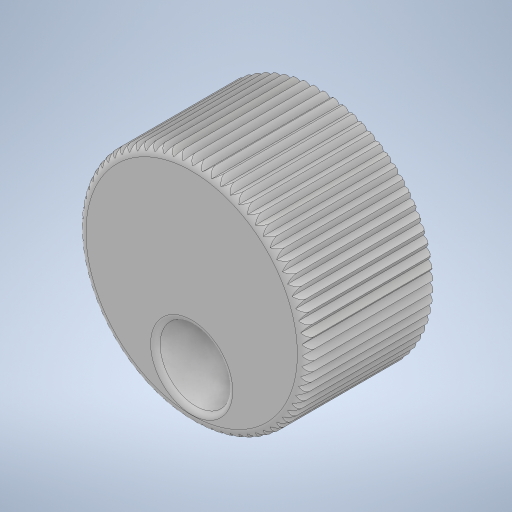
# Autodesk Inventor part: Encoder Knob
Saved by Autodesk Inventor 2024 (Build 280153000, 153)
## iProperties
Created: 2025-11-01
Part Number: Encoder Knob
Material: Generic
Document SubType Name: Modeling
Designer: Martin
Density: 1 g/cm^3
Appearance: Default
Author: Martin
Autodesk Inventor part; units mm, degrees
sketch "Sketch1" plane through (0, 0, 0) normal (0, 0, 1) x (1, 0, 0)
  circle A0 centre (0, 0) radius 15.875
  dimension "d0" = 31.75
  constraints: 1 centre point, 1 coincident
  measures "d0" diameter of A0
extrude "Extrusion1" add sketch "Sketch1" along normal blind 2.54
sketch "Sketch2" plane through (0, 0, 0) normal (0, 0, -1) x (-1, 0, 0)
  circle A0 centre (0, 0) radius 3.005
  circle A1 centre (0, 0) radius 5.08
  line L0 (0.7937, -5.0176) -> (0.7937, -2.8983)
  line L1 (-0.7937, -5.0176) -> (-0.7937, -2.8983)
  line L2 (-0.7937, -2.8983) -> (0.7937, -2.8983) construction
  line L3 (-2.6067, -1.495) -> (2.6067, -1.495) construction
  line L4 (2.5097, -1.6527) -> (2.1715, -1.495)
  line L5 (0.3685, -1.495) -> (1.9904, -2.2513)
  line L6 (0.3685, -1.495) -> (2.1715, -1.495)
  line L7 (0, -1.495) -> (0, -2.8983) construction
  line L8 (-2.5097, -1.6527) -> (-2.1715, -1.495)
  line L9 (-0.3685, -1.495) -> (-1.9904, -2.2513)
  line L10 (-0.3685, -1.495) -> (-2.1715, -1.495)
  point P0 (1.27, -1.495)
  point P1 (-1.27, -1.495)
  point P2 (-2.5097, -1.6527)
  point P3 (-1.9904, -2.2513)
  dimension "d3" = 6.01
  dimension "d4" = 10.16
  dimension "d5" = 1.5875
  dimension "d6" = 4.5
  dimension "d7" = 0.762
  dimension "d9" = 1.27
  dimension "d10" = 25
  constraints: 22 end point, 8 point on circle, 5 symmetric about line, 3 midpoint, 2 centre point, 2 coincident, 2 horizontal, 2 parallel, 2 point on line, 1 collinear, 1 vertical
  measures "d3" diameter of A0
  measures "d4" diameter of A1
  measures "d5" distance between parallel lines of L0 L1
  measures "d7" distance between parallel lines of L5 L4
  measures "d9" distance of L7.start point (1.27, -1.495)
  measures "d10" angle of L5 L3
extrude "Extrusion2" add sketch "Sketch2" along normal blind 6.35 contours A0 L1 A1 L0 | L8 L10 L9 A0 | A0 L5 L6 L4 picked at (4.3399, 0.4021)
sketch "Sketch3" plane through (0, 0, 0) normal (0, 0, -1) x (-1, 0, 0)
  circle A0 centre (0, 0) radius 15.875 projected
  circle A1 centre (0, 0) radius 13.335
  dimension "d13" = 2.54
  constraints: 1 centre point
  measures "d13" radial gap between concentric circles of A0 A1
extrude "Extrusion3" add sketch "Sketch3" along normal blind 15.24
ref_plane "Work Plane2" through (0, 0, 3.175) normal (0, 0, 1) x (1, 0, 0)
sketch "Sketch5" plane through (0, 0, 3.175) normal (0, 0, 1) x (1, 0, 0)
  arc A0 (0, -2.54) -> (0, -15.24) centre (0, -8.89) ccw
  line L0 (0, -15.24) -> (0, -2.54)
  point P0 (0, 0)
  point P1 (0, -3.81)
  point P2 (0, -13.97)
  dimension "d24" = 8.89
  dimension "d25" = 6.35
  constraints: 2 end point, 2 point on circle, 2 point on line, 2 vertical alignment, 1 centre point, 1 coincident, 1 midpoint, 1 vertical
  measures "d24" distance of point (0, 0) point (0, -8.89)
  measures "d25" radius of A0
revolve "Revolution2" add sketch "Sketch5" angle 180 about axis through (0, -15.24, 3.175) along (0, -1, 0)
sketch "Sketch7" plane through (0, 0, 3.175) normal (0, 0, 1) x (1, 0, 0)
  circle A0 centre (0, -8.89) radius 6.35 projected
  arc A1 (0, -3.81) -> (0, -13.97) centre (0, -8.89) ccw
  line L0 (0, -13.97) -> (0, -3.81)
  point P0 (0, 0)
  point P1 (0, -8.89)
  dimension "d28" = 5.08
  constraints: 2 coincident, 2 end point, 2 point on circle, 1 centre point, 1 midpoint, 1 vertical
  measures "d28" radius of A1
revolve "Revolution3" cut sketch "Sketch7" angle 180 about axis through (0, -13.97, 3.175) along (0, -1, 0) contours L0 A1
ref_plane "Work Plane3" through (0, 0, 2.54) normal (0, 0, 1) x (1, 0, 0)
split "Split1" plane through (0, 0, 2.54) removes the side toward (0, 0, 1)
fillet "Fillet1" radius 0.762 1 edges at (0, -3.8498, 2.54)
fillet "Fillet2" radius 1.27 1 edges at (-15.875, 0, 2.54)
fillet "Fillet4" radius 0.0508 2 edges at (-0.3685, -1.495, -3.175) (0.3685, -1.495, -3.175)
fillet "Fillet5" radius 0.508 1 edges at (15.875, 0, -15.24)
fillet "Fillet6" radius 0.254 1 edges at (0, 3.005, -6.35)
ref_plane "Work Plane4" through (0, 0, -6.35) normal (0, 0, 1) x (1, 0, 0)
sketch "Sketch8" plane through (0, 0, -6.35) normal (0, 0, 1) x (1, 0, 0)
  circle A0 centre (0, 0) radius 15.875 projected
  line L0 (0, -15.162) -> (0.6977, -15.8597)
  line L1 (0, -15.162) -> (0.9867, -15.162) construction
  line L2 (0, -15.162) -> (-0.6977, -15.8597)
  dimension "d40" = 45
  constraints: 6 end point, 2 point on circle, 1 equal length, 1 horizontal
  measures "d40" angle of L0 L1
extrude "Extrusion4" cut sketch "Sketch8" along normal through all both and the other way through all contours L2 L0 A0 picked at (-0.3101, -15.6317)
pattern_circular "Circular Pattern1" count 72 over 360 about axis through (0, 0, -10) along (0, 0, 1) of "Extrusion4"
body "Solid1"
